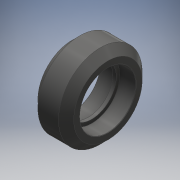
# Autodesk Inventor part: Solid V Wheel
Saved by Autodesk Inventor 2016 (Build 200138000, 138)
## iProperties
Created: 2016-10-20
Part Number: Solid V Wheel
Material: Типовые
Document SubType Name: Modeling
Designer: skhalipa
Density: 1 g/cm^3
Appearance: Темно-серый
Mass: 2.24975 g
Surface Area: 16.6137 cm^2
Volume: 2.24975 cm^3
Author: skhalipa
Autodesk Inventor part; units mm, degrees
ref_plane "YZ Plane" through (0, 0, 0) normal (1, 0, 0) x (0, 1, 0)
ref_plane "XZ Plane" through (0, 0, 0) normal (0, 1, 0) x (-1, 0, 0)
ref_plane "XY Plane" through (0, 0, 0) normal (0, 0, 1) x (1, 0, 0)
sketch "Эскиз4" plane through (0, 0, 0) normal (0, 0, 1) x (1, 0, 0)
  line L0 (-5.115, 7.987) -> (-5.115, 9.77)
  line L1 (-5.115, 9.77) -> (-2.945, 11.945)
  line L2 (-2.945, 11.945) -> (2.945, 11.945)
  line L3 (2.945, 11.945) -> (5.115, 9.77)
  line L4 (5.115, 9.77) -> (5.115, 7.987)
  line L5 (5.115, 7.987) -> (0.5, 7.987)
  line L6 (0.5, 7.987) -> (0.5, 6.987)
  line L7 (0.5, 6.987) -> (-0.5, 6.987)
  line L8 (-0.5, 6.987) -> (-0.5, 7.987)
  line L9 (-0.5, 7.987) -> (-5.115, 7.987)
  line L10 (-5.115, 0) -> (5.115, 0)
  point P0 (0, 0)
  point P1 (0, 11.945)
  point P2 (0, 6.987)
  point P3 (0, 0)
  dimension "d18" = 10.23
  dimension "d19" = 5.89
  dimension "d20" = 1
  dimension "d21" = 1
  dimension "d22" = 11.945
  dimension "d23" = 9.77
  dimension "d24" = 7.987
  dimension "d25" = 2.17
  dimension "d26" = 4.615
  dimension "d27" = 7.987
  constraints: 22 end point, 6 vertical alignment, 4 horizontal alignment, 3 midpoint, 3 perpendicular, 2 parallel, 1 horizontal, 1 point on line, 1 vertical
  measures "d18" distance between parallel lines of L4 L0
  measures "d19" distance of L1.end L2.end
  measures "d20" distance of L6.end L7.end
  measures "d21" distance of L5.end L6.end
  measures "d22" distance from line of point (0, 0) L2
  measures "d23" vertical distance of point (0, 0) L3.end
  measures "d24" vertical distance of point (0, 0) L4.end
  measures "d25" horizontal distance of L1.end L0.end
  measures "d26" distance of L4.end L5.end
  measures "d27" distance between parallel lines of L10 L9
revolve "Вращение1" add sketch "Эскиз4" angle 360 about axis through (-5.115, 0, 0) along (1, 0, 0)
chamfer "Фаска1" distance 0.1 angle 45 2 edges at (5.115, -7.987, 0) (-5.115, -7.987, 0)
